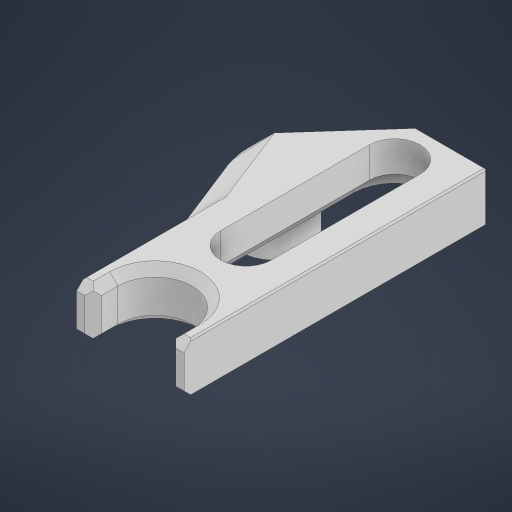
# Autodesk Inventor part: Halterrung_Stange
Saved by Autodesk Inventor 2024.2 (Build 282272000, 272)
## iProperties
Created: 2024-02-24
Part Number: Halterrung_Stange
Material: Generisch
Document SubType Name: Modeling
Designer: jacob
Density: 1 g/cm^3
Appearance: Vorgabe
Author: jacob
Autodesk Inventor part; units mm, degrees
ref_plane "YZ Plane" through (0, 0, 0) normal (1, 0, 0) x (0, 1, 0)
ref_plane "XZ Plane" through (0, 0, 0) normal (0, 1, 0) x (-1, 0, 0)
sketch "Skizze2" plane through (0, 0, 0) normal (0, 1, 0) x (-1, 0, 0)
  line L0 (0, -30) -> (6.5, -30)
  line L1 (6.5, -30) -> (6.5, 7.5)
  line L2 (6.5, 7.5) -> (4.5, 7.5)
  line L3 (4.5, 7.5) -> (4.5, 4.5)
  arc A0 (0, 0) -> (4.5, 4.5) centre (0, 4.5) ccw
  line L4 (0, 0) -> (0, -30)
  dimension "d16" = 2
  dimension "d17" = 3
  dimension "d18" = 30
  dimension "d19" = 4.5
  constraints: 10 end point, 3 perpendicular, 2 point on circle, 1 centre point, 1 coincident, 1 horizontal, 1 parallel, 1 tangent, 1 vertical alignment
  measures "d16" distance of L1.end L2.end
  measures "d17" distance of L2.end L3.end
  measures "d18" distance of L4.start L0.start
  measures "d19" radius of A0
extrude "Extrusion1" add sketch "Skizze2" along normal blind 6
mirror "Spiegeln1" about plane through (0, 0, 0) normal (1, 0, 0) of "Extrusion1"
sketch "Skizze3" plane through (0, 6, 0) normal (0, 1, 0) x (1, 0, 0)
  line L0 (3.075, 6.5) -> (3.075, 24.5)
  arc A0 (3.075, 24.5) -> (-3.075, 24.5) centre (0, 24.5) ccw
  line L1 (-3.075, 24.5) -> (-3.075, 6.5)
  arc A1 (-3.075, 6.5) -> (3.075, 6.5) centre (0, 6.5) ccw
  line L2 (-6.5, 30) -> (6.5, 30) projected
  arc A2 (4.5, -4.5) -> (-4.5, -4.5) centre (0, -4.5) ccw projected
  line L3 (6.5, -7.5) -> (4.5, -7.5) projected
  point P0 (0, 0)
  point P1 (0, 30)
  point P2 (0, 0)
  dimension "d8" = 6.15
  dimension "d11" = 18
  dimension "d15" = 14
  constraints: 5 point on circle, 4 end point, 4 tangent, 2 centre point, 1 midpoint, 1 parallel, 1 vertical, 1 vertical alignment
  measures "d8" distance between parallel lines of L1 L0
  measures "d11" distance of A0.centre A1.centre
  measures "d15" distance from line of L3 A1.centre
extrude "Extrusion2" cut sketch "Skizze3" along normal through all both and the other way through all
chamfer "Fasen1" distance 1 angle 45 6 edges at (-4.5, 3, 7.5) (4.5, 3, 7.5) (-5.5, 0, 7.5) (-5.5, 6, 7.5) (5.5, 6, 7.5) (5.5, 0, 7.5)
chamfer "Fasen2" distance 1 angle 45 1 edges at (6.5, 3, -30)
sketch "Skizze8" plane through (0, 0, 0) normal (0, -1, 0) x (1, 0, 0)
  circle A0 centre (-10.075, -20) radius 4
  line L0 (-3.075, -24.5) -> (-3.075, -6.5) projected
  line L1 (-6.5, -30) -> (-6.5, 6.5) projected
  line L2 (-6.5, 0) -> (-13.7969, -18.5347)
  line L3 (-6.5, -30) -> (-13.057, -22.6661)
  arc A1 (-4.5, 4.5) -> (4.5, 4.5) centre (0, 4.5) ccw projected
  point P0 (0, 0)
  point P1 (0, 0)
  point P2 (-6.5, -21.7943)
  point P3 (-6.5, -18.2057)
  dimension "d55" = 8
  dimension "d59" = 4.5
  dimension "d60" = 7
  dimension "d72" = 0
  constraints: 4 end point, 3 point on circle, 2 tangent, 1 centre point, 1 point on line
  measures "d55" diameter of A0
  measures "d59" vertical distance of L0.start A0.centre
  measures "d60" distance from line of L0 A0.centre
  measures "d72" vertical distance of point (0, 0) L2.start
extrude "Extrusion5" add sketch "Skizze8" against normal up to surface (6 mm away)
sketch "Skizze9" plane through (0, 0, 0) normal (0, -1, 0) x (1, 0, 0)
  circle A0 centre (-10.075, -20) radius 4
  arc A1 (-13.7969, -18.5347) -> (-13.057, -22.6661) centre (-10.075, -20) ccw projected
  point P0 (0, 0)
  point P1 (-7.5, -15.7292)
  point P2 (-7.5, -24.2708)
  constraints: 2 concentric, 1 centre point
extrude "Extrusion6" add sketch "Skizze9" along normal blind 4.5
sketch "Skizze10" plane through (-10.075, -4.5, -20) normal (0, -1, 0) x (1, 0, 0)
  circle A0 centre (0, 0) radius 4 projected
  point P0 (10.075, 20)
  constraints: 1 coincident
hole "Bohrung3" at (-10.075, -4.5, -20) direction (0, 1, 0) diameter 5.2 depth 2.5
chamfer "Fasen3" distance 4 angle 45 3 edges at (-9.7785, 6, -26.333) (-14.0123, 6, -20.7052) (-10.1485, 6, -9.2674)
chamfer "Fasen4" distance 1 angle 45 6 edges at (0, 6, 0) (4.5, 6, 5.5) (-4.5, 6, 5.5) (0, 0, 0) (4.5, 0, 5.5) (-4.5, 0, 5.5)
chamfer "Fasen5" distance 0.2 angle 45 5 edges at (-6.5, 6, -5.4596) (-6.5, 6, 3.25) (6.5, 6, -11.25) (6.5, 0, -11.25) (-6.5, 0, 3.25)
chamfer "Fasen6" distance 1 angle 45 1 edges at (2.1828, 6, -30)
sketch "Skizze11" plane through (-10.075, -4.5, -20) normal (0, -1, 0) x (1, 0, 0)
  circle A0 centre (0, 0) radius 4 projected
  point P0 (10.075, 20)
  point P1 (-4, 0)
  constraints: 1 horizontal alignment, 1 other
ref_plane "Arbeitsebene1" through (-14.075, -4.5, -20) normal (-1, 0, 0) x (0, -1, 0)
sketch "Skizze12" plane through (-14.075, -4.5, -20) normal (-1, 0, 0) x (0, -1, 0)
  line L0 (-2.5, 2.6) -> (0, 2.6) projected
  line L1 (0, 2.6) -> (-10.5, 2.6)
  line L2 (0, -4) -> (0, 4) projected
  line L3 (0, 2.6) -> (0, -2.6) projected
  line L4 (0, -2.6661) -> (-10.5, -2.6661)
  line L5 (-10.5, 9.5887) -> (-10.5, 0) projected
  line L6 (-10.5, 0) -> (-10.5, -9) projected
  line L7 (-4.5, -2.6661) -> (-6.5, -2.6661) projected
  point P0 (-4.5, 20)
  constraints: 4 end point, 3 point on line, 2 perpendicular, 1 collinear, 1 horizontal
extrude "Extrusion7" cut sketch "Skizze12" against normal blind 0.5
chamfer "Fasen7" distance 0.2 angle 45 1 edges at (-10.075, -4.5, -17.4)
sketch "Skizze13" plane through (0, 0, 0) normal (0, -1, 0) x (1, 0, 0)
  line L0 (5, -24.5) -> (5, -6.5)
  line L1 (-5, -24.5) -> (-5, -6.5)
  arc A0 (5, -6.5) -> (-5, -6.5) centre (0, -6.5) ccw
  arc A1 (3.075, -6.5) -> (-3.075, -6.5) centre (0, -6.5) ccw projected
  arc A2 (-5, -24.5) -> (5, -24.5) centre (0, -24.5) ccw
  arc A3 (-3.075, -24.5) -> (3.075, -24.5) centre (0, -24.5) ccw projected
  point P0 (0, 0)
  dimension "d90" = 10
  dimension "d91" = 0
  constraints: 4 end point, 4 point on circle, 2 centre point, 2 horizontal alignment, 2 tangent, 2 vertical, 1 concentric
  measures "d90" distance between parallel lines of L1 L0
  measures "d91" distance of A2.centre A3.centre
extrude "Extrusion8" cut sketch "Skizze13" against normal blind 2.3
